Autodesk Fusion 360 part; units mm, degrees
note: some values were not read from the file. Set by a fixed rule: which sketch regions a step uses.
(part 3 of 5)
  spline S639 degree 3 poles (-6.513678, -34.419833) (-6.519277, -34.39743) (-6.526746, -34.375961) (-6.536703, -34.354802) knots 0 0 0 0 1 1 1 1
  spline S640 degree 3 poles (-6.536703, -34.354802) (-6.546349, -34.333955) (-6.557862, -34.314042) (-6.571552, -34.295373) knots 0 0 0 0 1 1 1 1
  spline S641 degree 3 poles (-6.571552, -34.295373) (-6.585243, -34.276704) (-6.600489, -34.25959) (-6.617603, -34.244033) knots 0 0 0 0 1 1 1 1
  spline S642 degree 3 poles (-6.617603, -34.244033) (-6.634404, -34.228475) (-6.652762, -34.214474) (-6.672365, -34.20265) knots 0 0 0 0 1 1 1 1
  spline S643 degree 3 poles (-6.672365, -34.20265) (-6.692279, -34.190515) (-6.712815, -34.180558) (-6.734595, -34.172779) knots 0 0 0 0 1 1 1 1
  spline S644 degree 3 poles (-6.734595, -34.172779) (-6.756065, -34.164689) (-6.778467, -34.159089) (-6.801181, -34.155355) knots 0 0 0 0 1 1 1 1
  spline S645 degree 3 poles (-6.801181, -34.155355) (-6.823895, -34.15193) (-6.84692, -34.150688) (-6.869946, -34.151619) knots 0 0 0 0 1 1 1 1
  spline S646 degree 3 poles (-6.869946, -34.151619) (-6.892971, -34.15255) (-6.915684, -34.155666) (-6.938087, -34.161264) knots 0 0 0 0 1 1 1 1
  spline S647 degree 3 poles (-6.938087, -34.161264) (-6.96049, -34.166554) (-6.98227, -34.174333) (-7.003117, -34.183978) knots 0 0 0 0 1 1 1 1
  spline S648 degree 3 poles (-7.003117, -34.183978) (-7.024276, -34.193624) (-7.043878, -34.205448) (-7.062547, -34.218827) knots 0 0 0 0 1 1 1 1
  spline S649 degree 3 poles (-7.062547, -34.218827) (-7.081217, -34.232518) (-7.098329, -34.247764) (-7.114198, -34.264877) knots 0 0 0 0 1 1 1 1
  spline S650 degree 3 poles (-7.114198, -34.264877) (-7.752679, -34.978656) (-8.346665, -35.728217) (-8.895845, -36.513561) knots 0 0 0 0 1 1 1 1
  spline S651 degree 3 poles (-8.895845, -36.513561) (-8.903935, -36.454753) (-8.912647, -36.395946) (-8.921671, -36.337761) knots 0 0 0 0 1 1 1 1
  line L13 (-8.921671, -36.337761) -> (-9.100893, -34.942252)
  spline S652 degree 3 poles (-9.100893, -34.942252) (-9.103697, -34.919227) (-9.108983, -34.896824) (-9.116451, -34.874732) knots 0 0 0 0 1 1 1 1
  spline S653 degree 3 poles (-9.116451, -34.874732) (-9.123604, -34.852951) (-9.132942, -34.831793) (-9.144454, -34.811569) knots 0 0 0 0 1 1 1 1
  spline S654 degree 3 poles (-9.144454, -34.811569) (-9.155967, -34.791655) (-9.169346, -34.772675) (-9.184593, -34.75525) knots 0 0 0 0 1 1 1 1
  spline S655 degree 3 poles (-9.184593, -34.75525) (-9.199528, -34.737826) (-9.21633, -34.721957) (-9.234688, -34.707955) knots 0 0 0 0 1 1 1 1
  spline S656 degree 3 poles (-9.234688, -34.707955) (-9.253046, -34.693643) (-9.272337, -34.681508) (-9.293184, -34.67124) knots 0 0 0 0 1 1 1 1
  spline S657 degree 3 poles (-9.293184, -34.67124) (-9.31372, -34.660972) (-9.335501, -34.652571) (-9.357592, -34.646659) knots 0 0 0 0 1 1 1 1
  spline S658 degree 3 poles (-9.357592, -34.646659) (-9.379995, -34.640438) (-9.402709, -34.636702) (-9.425734, -34.635146) knots 0 0 0 0 1 1 1 1
  spline S659 degree 3 poles (-9.425734, -34.635146) (-9.448759, -34.633593) (-9.471784, -34.634215) (-9.494809, -34.637322) knots 0 0 0 0 1 1 1 1
  spline S660 degree 3 poles (-9.494809, -34.637322) (-9.517835, -34.640125) (-9.540237, -34.645412) (-9.562018, -34.652568) knots 0 0 0 0 1 1 1 1
  spline S661 degree 3 poles (-9.562018, -34.652568) (-9.58411, -34.660031) (-9.604957, -34.669682) (-9.625181, -34.681194) knots 0 0 0 0 1 1 1 1
  spline S662 degree 3 poles (-9.625181, -34.681194) (-9.645095, -34.692707) (-9.663764, -34.706086) (-9.681189, -34.721332) knots 0 0 0 0 1 1 1 1
  spline S663 degree 3 poles (-9.681189, -34.721332) (-9.698613, -34.736268) (-9.714482, -34.75307) (-9.728483, -34.771428) knots 0 0 0 0 1 1 1 1
  spline S664 degree 3 poles (-9.728483, -34.771428) (-9.742796, -34.789786) (-9.754931, -34.809388) (-9.765199, -34.830235) knots 0 0 0 0 1 1 1 1
  spline S665 degree 3 poles (-9.765199, -34.830235) (-9.775467, -34.850771) (-9.783557, -34.872552) (-9.78978, -34.894954) knots 0 0 0 0 1 1 1 1
  spline S666 degree 3 poles (-9.78978, -34.894954) (-9.795691, -34.917046) (-9.799426, -34.93976) (-9.800981, -34.963096) knots 0 0 0 0 1 1 1 1
  spline S667 degree 3 poles (-9.800981, -34.963096) (-9.802535, -34.986121) (-9.801914, -35.009147) (-9.799117, -35.032172) knots 0 0 0 0 1 1 1 1
  line L14 (-9.799117, -35.032172) -> (-9.614915, -36.433597)
  spline S668 degree 3 poles (-12.713349, -48.832314) (-12.663254, -48.841337) (-12.617515, -48.860318) (-12.575511, -48.888943) knots 0 0 0 0 1 1 1 1
  spline S669 degree 3 poles (-12.575511, -48.888943) (-12.093538, -49.210362) (-11.58294, -49.476706) (-11.043407, -49.688288) knots 0 0 0 0 1 1 1 1
  spline S670 degree 3 poles (-11.043407, -49.688288) (-10.504181, -49.89956) (-9.948468, -50.05109) (-9.376574, -50.142879) knots 0 0 0 0 1 1 1 1
  spline S671 degree 3 poles (-9.376574, -50.142879) (-8.808723, -50.255515) (-8.234962, -50.305922) (-7.656535, -50.294098) knots 0 0 0 0 1 1 1 1
  spline S672 degree 3 poles (-7.656535, -50.294098) (-7.077172, -50.282586) (-6.5059, -50.209154) (-5.942718, -50.073493) knots 0 0 0 0 1 1 1 1
  spline S673 degree 3 poles (-5.943652, -50.073493) (-5.920315, -50.066961) (-5.89729, -50.062602) (-5.873954, -50.060735) knots 0 0 0 0 1 1 1 1
  spline S674 degree 3 poles (-5.874575, -50.060738) (-5.850306, -50.058871) (-5.82697, -50.059182) (-5.803634, -50.061978) knots 0 0 0 0 1 1 1 1
  spline S675 degree 3 poles (-5.804566, -50.061669) (-5.780297, -50.06478) (-5.757583, -50.069759) (-5.73518, -50.076913) knots 0 0 0 0 1 1 1 1
  spline S676 degree 3 poles (-5.735802, -50.076915) (-5.712777, -50.084376) (-5.69162, -50.093715) (-5.671083, -50.105227) knots 0 0 0 0 1 1 1 1
  spline S677 degree 3 poles (-5.671705, -50.10523) (-5.650547, -50.117051) (-5.631567, -50.130431) (-5.613831, -50.145988) knots 0 0 0 0 1 1 1 1
  spline S678 degree 3 poles (-5.614454, -50.145991) (-5.596096, -50.161546) (-5.580228, -50.178348) (-5.565914, -50.197017) knots 0 0 0 0 1 1 1 1
  spline S679 degree 3 poles (-5.566536, -50.197019) (-5.551601, -50.215686) (-5.539155, -50.235599) (-5.528887, -50.256758) knots 0 0 0 0 1 1 1 1
  spline S680 degree 3 poles (-5.529509, -50.25676) (-5.518619, -50.277916) (-5.510529, -50.300008) (-5.504618, -50.322721) knots 0 0 0 0 1 1 1 1
  spline S681 degree 3 poles (-5.505239, -50.322724) (-5.498707, -50.345435) (-5.494972, -50.368461) (-5.493727, -50.392108) knots 0 0 0 0 1 1 1 1
  spline S682 degree 3 poles (-5.494349, -50.39211) (-5.492485, -50.415755) (-5.493409, -50.439092) (-5.496842, -50.462428) knots 0 0 0 0 1 1 1 1
  spline S683 degree 3 poles (-5.497464, -50.462119) (-5.500267, -50.485453) (-5.505866, -50.508167) (-5.513956, -50.53057) knots 0 0 0 0 1 1 1 1
  spline S684 degree 3 poles (-5.514577, -50.530261) (-5.521738, -50.552662) (-5.532002, -50.57382) (-5.544137, -50.593733) knots 0 0 0 0 1 1 1 1
  spline S685 degree 3 poles (-5.544758, -50.593736) (-5.556272, -50.613958) (-5.570274, -50.632627) (-5.586143, -50.650052) knots 0 0 0 0 1 1 1 1
  spline S686 degree 3 poles (-5.587075, -50.650054) (-5.602322, -50.667476) (-5.619746, -50.683034) (-5.638726, -50.696724) knots 0 0 0 0 1 1 1 1
  spline S687 degree 3 poles (-5.639348, -50.696415) (-5.657707, -50.710415) (-5.677931, -50.722238) (-5.699401, -50.731884) knots 0 0 0 0 1 1 1 1
  spline S688 degree 3 poles (-5.700022, -50.731887) (-5.72087, -50.741841) (-5.742962, -50.749309) (-5.765987, -50.754598) knots 0 0 0 0 1 1 1 1
  spline S689 degree 3 poles (-5.766608, -50.754289) (-6.378019, -50.903017) (-6.999075, -50.984227) (-7.628844, -50.997918) knots 0 0 0 0 1 1 1 1
  spline S690 degree 3 poles (-7.629154, -50.997609) (-8.258612, -51.011608) (-8.882468, -50.957779) (-9.500411, -50.836122) knots 0 0 0 0 1 1 1 1
  spline S691 degree 3 poles (-9.500411, -50.836122) (-10.12178, -50.735618) (-10.7251, -50.570086) (-11.310995, -50.339526) knots 0 0 0 0 1 1 1 1
  spline S692 degree 3 poles (-11.310995, -50.339526) (-11.896892, -50.108961) (-12.451362, -49.818658) (-12.974716, -49.468616) knots 0 0 0 0 1 1 1 1
  spline S693 degree 3 poles (-12.974716, -49.468616) (-13.007699, -49.4459) (-13.036013, -49.418208) (-13.059661, -49.385537) knots 0 0 0 0 1 1 1 1
  spline S694 degree 3 poles (-13.059661, -49.385537) (-13.082996, -49.353177) (-13.10042, -49.317706) (-13.111934, -49.279123) knots 0 0 0 0 1 1 1 1
  spline S695 degree 3 poles (-13.111934, -49.279123) (-13.123447, -49.240541) (-13.128114, -49.201336) (-13.125936, -49.161197) knots 0 0 0 0 1 1 1 1
  spline S696 degree 3 poles (-13.125936, -49.161197) (-13.124071, -49.121059) (-13.115357, -49.082165) (-13.10011, -49.045138) knots 0 0 0 0 1 1 1 1
  spline S697 degree 3 poles (-13.10011, -49.045138) (-13.084864, -49.008112) (-13.063706, -48.974507) (-13.036947, -48.944326) knots 0 0 0 0 1 1 1 1
  spline S698 degree 3 poles (-13.036947, -48.944326) (-13.010188, -48.914455) (-12.979384, -48.889874) (-12.944224, -48.870583) knots 0 0 0 0 1 1 1 1
  spline S699 degree 3 poles (-12.944224, -48.870583) (-12.909064, -48.850981) (-12.871415, -48.838223) (-12.831899, -48.831689) knots 0 0 0 0 1 1 1 1
  spline S700 degree 3 poles (-12.831899, -48.831689) (-12.792383, -48.825158) (-12.752867, -48.825158) (-12.713349, -48.832314) knots 0 0 0 0 1 1 1 1
  spline S701 degree 3 poles (-13.602617, -45.813223) (-13.50616, -45.830336) (-13.43024, -45.879498) (-13.374544, -45.959782) knots 0 0 0 0 1 1 1 1
  spline S702 degree 3 poles (-13.374544, -45.959782) (-13.314803, -46.051253) (-13.252573, -46.140553) (-13.188165, -46.228608) knots 0 0 0 0 1 1 1 1
  spline S703 degree 3 poles (-13.187853, -46.227682) (-13.123445, -46.316353) (-13.056859, -46.402541) (-12.988095, -46.486863) knots 0 0 0 0 1 1 1 1
  spline S704 degree 3 poles (-12.988095, -46.486248) (-12.919331, -46.571185) (-12.848388, -46.653951) (-12.775268, -46.73485) knots 0 0 0 0 1 1 1 1
  spline S705 degree 3 poles (-12.775268, -46.733924) (-12.702148, -46.815438) (-12.627161, -46.89447) (-12.550307, -46.971324) knots 0 0 0 0 1 1 1 1
  spline S706 degree 3 poles (-12.549995, -46.970709) (-12.473141, -47.048489) (-12.394109, -47.123477) (-12.313521, -47.196597) knots 0 0 0 0 1 1 1 1
  spline S707 degree 3 poles (-12.31321, -47.195671) (-12.232622, -47.269406) (-12.149856, -47.340348) (-12.065534, -47.409113) knots 0 0 0 0 1 1 1 1
  spline S708 degree 3 poles (-12.065534, -47.408498) (-11.981213, -47.477877) (-11.895024, -47.544774) (-11.80728, -47.609182) knots 0 0 0 0 1 1 1 1
  spline S709 degree 3 poles (-11.80728, -47.608256) (-11.719535, -47.67359) (-11.630235, -47.73582) (-11.539068, -47.795561) knots 0 0 0 0 1 1 1 1
  spline S710 degree 3 poles (-11.539068, -47.794946) (-11.448212, -47.855613) (-11.355801, -47.913176) (-11.261833, -47.96825) knots 0 0 0 0 1 1 1 1
  spline S711 degree 3 poles (-11.261833, -47.967635) (-11.168177, -48.023323) (-11.072965, -48.076219) (-10.976508, -48.126625) knots 0 0 0 0 1 1 1 1
  spline S712 degree 3 poles (-10.976197, -48.12601) (-10.879741, -48.177032) (-10.782039, -48.224949) (-10.683094, -48.270377) knots 0 0 0 0 1 1 1 1
  spline S713 degree 3 poles (-10.683094, -48.269762) (-10.584148, -48.315805) (-10.484269, -48.358743) (-10.383145, -48.398882) knots 0 0 0 0 1 1 1 1
  spline S714 degree 3 poles (-10.382834, -48.398267) (-10.282021, -48.439331) (-10.179964, -48.47698) (-10.076973, -48.51214) knots 0 0 0 0 1 1 1 1
  spline S715 degree 3 poles (-10.076662, -48.511525) (-9.973671, -48.5473) (-9.870058, -48.579971) (-9.7652, -48.609842) knots 0 0 0 0 1 1 1 1
  spline S716 degree 3 poles (-9.7652, -48.609227) (-9.660654, -48.639712) (-9.555174, -48.666782) (-9.449072, -48.691363) knots 0 0 0 0 1 1 1 1
  spline S717 degree 3 poles (-9.449072, -48.690748) (-9.342969, -48.715944) (-9.236556, -48.737724) (-9.129209, -48.757016) knots 0 0 0 0 1 1 1 1
  spline S718 degree 3 poles (-9.129209, -48.75609) (-9.022173, -48.775996) (-8.914515, -48.792487) (-8.806545, -48.806177) knots 0 0 0 0 1 1 1 1
  spline S719 degree 3 poles (-8.806235, -48.805562) (-8.698577, -48.819868) (-8.590296, -48.830758) (-8.481704, -48.838848) knots 0 0 0 0 1 1 1 1
  spline S720 degree 3 poles (-8.481394, -48.838233) (-8.373113, -48.846938) (-8.26421, -48.852539) (-8.155619, -48.855028) knots 0 0 0 0 1 1 1 1
  spline S721 degree 3 poles (-8.155309, -48.854413) (-8.046716, -48.857831) (-7.937813, -48.857512) (-7.828911, -48.85471) knots 0 0 0 0 1 1 1 1
  spline S722 degree 3 poles (-7.828912, -48.854095) (-7.720008, -48.851914) (-7.611417, -48.846309) (-7.502825, -48.837907) knots 0 0 0 0 1 1 1 1
  spline S723 degree 3 poles (-7.502827, -48.837292) (-7.394234, -48.829506) (-7.285954, -48.818305) (-7.177984, -48.804614) knots 0 0 0 0 1 1 1 1
  spline S724 degree 3 poles (-7.177985, -48.803688) (-7.070015, -48.790613) (-6.962357, -48.774122) (-6.855321, -48.75483) knots 0 0 0 0 1 1 1 1
  spline S725 degree 3 poles (-6.855322, -48.753904) (-6.748285, -48.735228) (-6.641561, -48.713447) (-6.535459, -48.688555) knots 0 0 0 0 1 1 1 1
  spline S726 degree 3 poles (-6.53546, -48.68794) (-6.429357, -48.663974) (-6.324187, -48.636282) (-6.21933, -48.606412) knots 0 0 0 0 1 1 1 1
  spline S727 degree 3 poles (-6.219332, -48.605797) (-6.114784, -48.57623) (-6.01086, -48.543559) (-5.907869, -48.508088) knots 0 0 0 0 1 1 1 1
  spline S728 degree 3 poles (-5.90787, -48.507473) (-5.804878, -48.472928) (-5.702821, -48.434968) (-5.601697, -48.394207) knots 0 0 0 0 1 1 1 1
  spline S729 degree 3 poles (-5.601698, -48.393592) (-5.500885, -48.353758) (-5.400694, -48.310819) (-5.301749, -48.26508) knots 0 0 0 0 1 1 1 1
  spline S730 degree 3 poles (-5.30175, -48.264465) (-5.202803, -48.219341) (-5.105101, -48.171424) (-5.008645, -48.120706) knots 0 0 0 0 1 1 1 1
  spline S731 degree 3 poles (-5.008646, -48.120091) (-4.912188, -48.0703) (-4.817287, -48.017404) (-4.72332, -47.962019) knots 0 0 0 0 1 1 1 1
  spline S732 degree 3 poles (-4.723321, -47.961093) (-4.629664, -47.906635) (-4.537252, -47.848761) (-4.446396, -47.788709) knots 0 0 0 0 1 1 1 1
  spline S733 degree 3 poles (-4.446086, -47.788094) (-4.35554, -47.728657) (-4.26624, -47.666115) (-4.178496, -47.601707) knots 0 0 0 0 1 1 1 1
  spline S734 degree 3 poles (-4.178186, -47.601092) (-4.140535, -47.578371) (-4.099463, -47.562814) (-4.055591, -47.555035) knots 0 0 0 0 1 1 1 1
  spline S735 degree 3 poles (-4.055278, -47.554425) (-4.011719, -47.547254) (-3.967847, -47.547874) (-3.924286, -47.556899) knots 0 0 0 0 1 1 1 1
  spline S736 degree 3 poles (-3.923972, -47.556289) (-3.880414, -47.565923) (-3.839964, -47.582414) (-3.802626, -47.606994) knots 0 0 0 0 1 1 1 1
  spline S737 degree 3 poles (-3.802624, -47.606384) (-3.765288, -47.631264) (-3.733862, -47.661757) (-3.708036, -47.698162) knots 0 0 0 0 1 1 1 1
  spline S738 degree 3 poles (-3.708034, -47.697551) (-3.682211, -47.734566) (-3.664164, -47.774393) (-3.653585, -47.817643) knots 0 0 0 0 1 1 1 1
  spline S739 degree 3 poles (-3.653272, -47.817033) (-3.642695, -47.861204) (-3.640517, -47.905076) (-3.646429, -47.94926) knots 0 0 0 0 1 1 1 1
  spline S740 degree 3 poles (-3.646426, -47.948339) (-3.652652, -47.993443) (-3.666653, -48.034826) (-3.688434, -48.074031) knots 0 0 0 0 1 1 1 1
  spline S741 degree 3 poles (-3.68812, -48.07311) (-3.710214, -48.112925) (-3.738218, -48.146529) (-3.773067, -48.174533) knots 0 0 0 0 1 1 1 1
  spline S742 degree 3 poles (-3.772753, -48.173922) (-3.870146, -48.245786) (-3.969092, -48.314861) (-4.069593, -48.381136) knots 0 0 0 0 1 1 1 1
  spline S743 degree 3 poles (-4.069591, -48.380526) (-4.170406, -48.447411) (-4.272774, -48.511197) (-4.376698, -48.572183) knots 0 0 0 0 1 1 1 1
  spline S744 degree 3 poles (-4.376385, -48.571573) (-4.480623, -48.633479) (-4.585791, -48.691976) (-4.692827, -48.747671) knots 0 0 0 0 1 1 1 1
  spline S745 degree 3 poles (-4.692514, -48.747061) (-4.799552, -48.803367) (-4.907832, -48.856574) (-5.017357, -48.90698) knots 0 0 0 0 1 1 1 1
  spline S746 degree 3 poles (-5.017043, -48.90637) (-5.126882, -48.957387) (-5.237339, -49.004682) (-5.349354, -49.049487) knots 0 0 0 0 1 1 1 1
  spline S747 degree 3 poles (-5.349352, -49.048877) (-5.461368, -49.094293) (-5.574315, -49.135987) (-5.688197, -49.175192) knots 0 0 0 0 1 1 1 1
  spline S748 degree 3 poles (-5.688195, -49.174271) (-5.802389, -49.214086) (-5.917203, -49.250179) (-6.033263, -49.283472) knots 0 0 0 0 1 1 1 1
  spline S749 degree 3 poles (-6.032949, -49.282862) (-6.14901, -49.316454) (-6.265692, -49.346947) (-6.382995, -49.374017) knots 0 0 0 0 1 1 1 1
  spline S750 degree 3 poles (-6.382993, -49.373407) (-6.500299, -49.401398) (-6.618225, -49.425668) (-6.737084, -49.447137) knots 0 0 0 0 1 1 1 1
  spline S751 degree 3 poles (-6.736771, -49.446216) (-6.855633, -49.468296) (-6.974492, -49.486653) (-7.093974, -49.5019) knots 0 0 0 0 1 1 1 1
  spline S752 degree 3 poles (-7.093972, -49.50129) (-7.213766, -49.517146) (-7.33356, -49.529281) (-7.453664, -49.538615) knots 0 0 0 0 1 1 1 1
  spline S753 degree 3 poles (-7.45335, -49.538005) (-7.573768, -49.54795) (-7.694183, -49.553862) (-7.814598, -49.556973) knots 0 0 0 0 1 1 1 1
  spline S754 degree 3 poles (-7.814284, -49.556363) (-7.935013, -49.560087) (-8.055428, -49.560398) (-8.175843, -49.557292) knots 0 0 0 0 1 1 1 1
  spline S755 degree 3 poles (-8.17553, -49.556682) (-8.296257, -49.554489) (-8.416674, -49.548268) (-8.536778, -49.539245) knots 0 0 0 0 1 1 1 1
  spline S756 degree 3 poles (-8.536464, -49.538635) (-8.656882, -49.530222) (-8.776673, -49.518087) (-8.896155, -49.50284) knots 0 0 0 0 1 1 1 1
  spline S757 degree 3 poles (-8.896154, -49.50223) (-9.015637, -49.487905) (-9.134807, -49.469547) (-9.253356, -49.448389) knots 0 0 0 0 1 1 1 1
  spline S758 degree 3 poles (-9.253354, -49.447779) (-9.371904, -49.427231) (-9.48983, -49.403272) (-9.607445, -49.375891) knots 0 0 0 0 1 1 1 1
  spline S759 degree 3 poles (-9.607132, -49.375281) (-9.724748, -49.348821) (-9.84143, -49.31864) (-9.957178, -49.285658) knots 0 0 0 0 1 1 1 1
  spline S760 degree 3 poles (-9.957176, -49.285047) (-10.072925, -49.252676) (-10.188051, -49.216582) (-10.301932, -49.178) knots 0 0 0 0 1 1 1 1
  spline S761 degree 3 poles (-10.301931, -49.177078) (-10.416124, -49.139106) (-10.529072, -49.097101) (-10.641086, -49.052606) knots 0 0 0 0 1 1 1 1
  spline S762 degree 3 poles (-10.640774, -49.051996) (-10.752789, -49.008112) (-10.863558, -48.960817) (-10.973083, -48.91041) knots 0 0 0 0 1 1 1 1
  spline S763 degree 3 poles (-10.973082, -48.9098) (-11.082608, -48.860315) (-11.190888, -48.80742) (-11.297613, -48.751724) knots 0 0 0 0 1 1 1 1
  spline S764 degree 3 poles (-11.297612, -48.750802) (-11.404649, -48.696028) (-11.510129, -48.637532) (-11.614053, -48.576546) knots 0 0 0 0 1 1 1 1
  spline S765 degree 3 poles (-11.613741, -48.575936) (-11.717666, -48.515561) (-11.820034, -48.452086) (-11.920847, -48.385811) knots 0 0 0 0 1 1 1 1
  spline S766 degree 3 poles (-11.920535, -48.385201) (-12.021349, -48.319536) (-12.120294, -48.250772) (-12.217684, -48.179518) knots 0 0 0 0 1 1 1 1
  spline S767 degree 3 poles (-12.217683, -48.178908) (-12.314763, -48.108265) (-12.410286, -48.034833) (-12.503632, -47.958602) knots 0 0 0 0 1 1 1 1
  spline S768 degree 3 poles (-12.50363, -47.957991) (-12.597288, -47.882681) (-12.688766, -47.804271) (-12.778377, -47.723683) knots 0 0 0 0 1 1 1 1
  spline S769 degree 3 poles (-12.778065, -47.723073) (-12.867677, -47.643095) (-12.955111, -47.560018) (-13.040676, -47.475074) knots 0 0 0 0 1 1 1 1
  spline S770 degree 3 poles (-13.040365, -47.474153) (-13.125931, -47.389819) (-13.209009, -47.302697) (-13.289907, -47.213397) knots 0 0 0 0 1 1 1 1
  spline S771 degree 3 poles (-13.289907, -47.212475) (-13.371117, -47.124097) (-13.449527, -47.032618) (-13.52607, -46.939273) knots 0 0 0 0 1 1 1 1
  spline S772 degree 3 poles (-13.525759, -46.938663) (-13.602303, -46.845928) (-13.676045, -46.750716) (-13.747609, -46.653948) knots 0 0 0 0 1 1 1 1
  spline S773 degree 3 poles (-13.747609, -46.653027) (-13.819174, -46.55687) (-13.888249, -46.457924) (-13.954835, -46.357422) knots 0 0 0 0 1 1 1 1
  spline S774 degree 3 poles (-13.954524, -46.356812) (-13.974127, -46.328796) (-13.989062, -46.297993) (-13.99933, -46.265011) knots 0 0 0 0 1 1 1 1
  spline S775 degree 3 poles (-13.99933, -46.265011) (-14.009598, -46.232029) (-14.014887, -46.198113) (-14.015198, -46.163576) knots 0 0 0 0 1 1 1 1
  spline S776 degree 3 poles (-14.015198, -46.163576) (-14.015835, -46.129038) (-14.011152, -46.095123) (-14.001508, -46.061829) knots 0 0 0 0 1 1 1 1
  spline S777 degree 3 poles (-14.001508, -46.061829) (-13.991862, -46.028536) (-13.977549, -45.997421) (-13.95888, -45.968484) knots 0 0 0 0 1 1 1 1
  spline S778 degree 3 poles (-13.95888, -45.968484) (-13.9399, -45.939547) (-13.917497, -45.913722) (-13.891049, -45.891319) knots 0 0 0 0 1 1 1 1
  spline S779 degree 3 poles (-13.891049, -45.891319) (-13.864913, -45.868916) (-13.835665, -45.85087) (-13.804239, -45.837179) knots 0 0 0 0 1 1 1 1
  spline S780 degree 3 poles (-13.804239, -45.837179) (-13.772501, -45.823177) (-13.739519, -45.814465) (-13.705293, -45.810109) knots 0 0 0 0 1 1 1 1
  spline S781 degree 3 poles (-13.705293, -45.810109) (-13.670755, -45.806061) (-13.63684, -45.806995) (-13.602617, -45.813223) knots 0 0 0 0 1 1 1 1
  spline S782 degree 3 poles (-13.428991, -40.838231) (-13.406281, -40.842288) (-13.384189, -40.848509) (-13.362716, -40.8569) knots 0 0 0 0 1 1 1 1
  spline S783 degree 3 poles (-13.362716, -40.8569) (-13.341251, -40.865311) (-13.320715, -40.87589) (-13.301109, -40.888326) knots 0 0 0 0 1 1 1 1
  spline S784 degree 3 poles (-13.301109, -40.888326) (-13.281821, -40.900782) (-13.263774, -40.915095) (-13.246968, -40.930954) knots 0 0 0 0 1 1 1 1
  spline S785 degree 3 poles (-13.246968, -40.930954) (-13.230481, -40.946832) (-13.215546, -40.964568) (-13.202474, -40.983538) knots 0 0 0 0 1 1 1 1
  spline S786 degree 3 poles (-13.202474, -40.983538) (-13.189099, -41.002217) (-13.177897, -41.022442) (-13.168558, -41.04359) knots 0 0 0 0 1 1 1 1
  spline S787 degree 3 poles (-13.168558, -41.04359) (-13.159539, -41.064758) (-13.152382, -41.086539) (-13.1474, -41.109243) knots 0 0 0 0 1 1 1 1
  spline S788 degree 3 poles (-13.1474, -41.109243) (-13.142426, -41.131656) (-13.139622, -41.154681) (-13.13931, -41.177696) knots 0 0 0 0 1 1 1 1
  spline S789 degree 3 poles (-13.13931, -41.177696) (-13.138996, -41.200731) (-13.140556, -41.223756) (-13.1446, -41.24646) knots 0 0 0 0 1 1 1 1
  spline S790 degree 3 poles (-13.1446, -41.24646) (-13.162339, -41.345105) (-13.176963, -41.444362) (-13.188783, -41.543609) knots 0 0 0 0 1 1 1 1
  spline S791 degree 3 poles (-13.188783, -41.543609) (-13.200611, -41.643187) (-13.209634, -41.742755) (-13.215542, -41.842624) knots 0 0 0 0 1 1 1 1
  spline S792 degree 3 poles (-13.215542, -41.842624) (-13.222078, -41.942824) (-13.225503, -42.043015) (-13.226125, -42.143205) knots 0 0 0 0 1 1 1 1
  spline S793 degree 3 poles (-13.22581, -42.142573) (-13.226443, -42.243396) (-13.22426, -42.343275) (-13.218972, -42.443465) knots 0 0 0 0 1 1 1 1
  spline S794 degree 3 poles (-13.218657, -42.442833) (-13.213994, -42.543344) (-13.205904, -42.643224) (-13.195012, -42.742792) knots 0 0 0 0 1 1 1 1
  spline S795 degree 3 poles (-13.194699, -42.741849) (-13.184123, -42.84236) (-13.170743, -42.941617) (-13.154253, -43.040563) knots 0 0 0 0 1 1 1 1
  spline S796 degree 3 poles (-13.154253, -43.040563) (-13.137761, -43.139197) (-13.118471, -43.237521) (-13.096379, -43.335222) knots 0 0 0 0 1 1 1 1
  spline S797 degree 3 poles (-13.096379, -43.335222) (-13.074287, -43.432923) (-13.049706, -43.530002) (-13.022014, -43.626147) knots 0 0 0 0 1 1 1 1
  spline S798 degree 3 poles (-13.022014, -43.626147) (-12.994322, -43.722604) (-12.96414, -43.817816) (-12.931158, -43.912406) knots 0 0 0 0 1 1 1 1
  spline S799 degree 3 poles (-12.931158, -43.912406) (-12.898176, -44.006995) (-12.862705, -44.100652) (-12.824434, -44.193063) knots 0 0 0 0 1 1 1 1
  spline S800 degree 3 poles (-12.824434, -44.193063) (-12.786162, -44.285786) (-12.74509, -44.376953) (-12.70184, -44.467187) knots 0 0 0 0 1 1 1 1
  spline S801 degree 3 poles (-12.70184, -44.467187) (-12.658279, -44.55742) (-12.612229, -44.646409) (-12.56369, -44.733842) knots 0 0 0 0 1 1 1 1
  spline S802 degree 3 poles (-12.56369, -44.733842) (-12.51515, -44.821587) (-12.464433, -44.907775) (-12.410915, -44.992408) knots 0 0 0 0 1 1 1 1
  spline S803 degree 3 poles (-12.410915, -44.992408) (-12.357397, -45.077041) (-12.301701, -45.160118) (-12.243516, -45.24164) knots 0 0 0 0 1 1 1 1
  spline S804 degree 3 poles (-12.243516, -45.24164) (-12.185642, -45.323161) (-12.124968, -45.402816) (-12.062427, -45.480914) knots 0 0 0 0 1 1 1 1
  spline S805 degree 3 poles (-12.062427, -45.480914) (-11.999885, -45.559013) (-11.934855, -45.635245) (-11.867958, -45.70961) knots 0 0 0 0 1 1 1 1
  spline S806 degree 3 poles (-11.867958, -45.70961) (-11.80106, -45.783975) (-11.731985, -45.856473) (-11.660731, -45.926793) knots 0 0 0 0 1 1 1 1
  spline S807 degree 3 poles (-11.660731, -45.926793) (-11.589789, -45.997113) (-11.516669, -46.065566) (-11.441682, -46.131841) knots 0 0 0 0 1 1 1 1
  spline S808 degree 3 poles (-11.441682, -46.131841) (-11.366694, -46.198116) (-11.28984, -46.262213) (-11.21143, -46.324132) knots 0 0 0 0 1 1 1 1
  spline S809 degree 3 poles (-11.21143, -46.324132) (-11.132709, -46.38605) (-11.052433, -46.445791) (-10.970289, -46.503043) knots 0 0 0 0 1 1 1 1
  spline S810 degree 3 poles (-10.970289, -46.503043) (-10.888456, -46.560295) (-10.804757, -46.615368) (-10.719813, -46.667953) knots 0 0 0 0 1 1 1 1
  spline S811 degree 3 poles (-10.719813, -46.667953) (-10.634558, -46.720537) (-10.548058, -46.770632) (-10.460003, -46.818238) knots 0 0 0 0 1 1 1 1
  spline S812 degree 3 poles (-10.460003, -46.818238) (-10.371947, -46.865844) (-10.282647, -46.910961) (-10.192102, -46.953589) knots 0 0 0 0 1 1 1 1
  spline S813 degree 3 poles (-10.192102, -46.953589) (-10.101557, -46.996216) (-10.010079, -47.036043) (-9.917045, -47.073381) knots 0 0 0 0 1 1 1 1
  spline S814 degree 3 poles (-9.917045, -47.073381) (-9.824322, -47.11072) (-9.730666, -47.145257) (-9.635765, -47.177306) knots 0 0 0 0 1 1 1 1
  spline S815 degree 3 poles (-9.635765, -47.177306) (-9.540865, -47.209354) (-9.445341, -47.238602) (-9.348885, -47.265361) knots 0 0 0 0 1 1 1 1
  spline S816 degree 3 poles (-9.348885, -47.265361) (-9.252428, -47.291809) (-9.155349, -47.315456) (-9.057648, -47.336615) knots 0 0 0 0 1 1 1 1
  spline S817 degree 3 poles (-9.057648, -47.336615) (-8.959636, -47.357773) (-8.861312, -47.37582) (-8.762678, -47.391377) knots 0 0 0 0 1 1 1 1
  spline S818 degree 3 poles (-8.762678, -47.391377) (-8.663732, -47.406623) (-8.564475, -47.419381) (-8.464907, -47.429026) knots 0 0 0 0 1 1 1 1
  spline S819 degree 3 poles (-8.464907, -47.429026) (-8.365339, -47.438983) (-8.265771, -47.445828) (-8.16558, -47.449873) knots 0 0 0 0 1 1 1 1
  spline S820 degree 3 poles (-8.16558, -47.449873) (-8.065701, -47.453921) (-7.965822, -47.455474) (-7.865631, -47.45361) knots 0 0 0 0 1 1 1 1
  spline S821 degree 3 poles (-7.865631, -47.45361) (-7.765752, -47.452056) (-7.665873, -47.4477) (-7.565995, -47.440541) knots 0 0 0 0 1 1 1 1
  spline S822 degree 3 poles (-7.565995, -47.440541) (-7.542659, -47.438358) (-7.519322, -47.438358) (-7.495986, -47.44086) knots 0 0 0 0 1 1 1 1
  spline S823 degree 3 poles (-7.495986, -47.44086) (-7.47265, -47.443344) (-7.449936, -47.448021) (-7.427533, -47.454861) knots 0 0 0 0 1 1 1 1
  spline S824 degree 3 poles (-7.427533, -47.454861) (-7.405441, -47.462023) (-7.383973, -47.471041) (-7.363437, -47.482243) knots 0 0 0 0 1 1 1 1
  spline S825 degree 3 poles (-7.363437, -47.482243) (-7.342901, -47.493755) (-7.323609, -47.506824) (-7.305874, -47.52207) knots 0 0 0 0 1 1 1 1
  spline S826 degree 3 poles (-7.305874, -47.52207) (-7.287827, -47.537005) (-7.271647, -47.553807) (-7.257023, -47.572165) knots 0 0 0 0 1 1 1 1
  spline S827 degree 3 poles (-7.257023, -47.572165) (-7.24271, -47.590834) (-7.229953, -47.610437) (-7.219374, -47.631284) knots 0 0 0 0 1 1 1 1
  spline S828 degree 3 poles (-7.219374, -47.631284) (-7.208795, -47.652131) (-7.200394, -47.673911) (-7.194172, -47.696314) knots 0 0 0 0 1 1 1 1
  spline S829 degree 3 poles (-7.194172, -47.696314) (-7.18795, -47.719028) (-7.183904, -47.742053) (-7.182036, -47.765389) knots 0 0 0 0 1 1 1 1
  spline S830 degree 3 poles (-7.182036, -47.765389) (-7.180483, -47.788726) (-7.181104, -47.812062) (-7.18421, -47.835398) knots 0 0 0 0 1 1 1 1
  spline S831 degree 3 poles (-7.18421, -47.835398) (-7.187014, -47.858735) (-7.1923, -47.881448) (-7.199768, -47.90354) knots 0 0 0 0 1 1 1 1
  spline S832 degree 3 poles (-7.199768, -47.90354) (-7.207231, -47.925943) (-7.216881, -47.947101) (-7.228705, -47.967326) knots 0 0 0 0 1 1 1 1
  spline S833 degree 3 poles (-7.228705, -47.967326) (-7.240529, -47.987551) (-7.254219, -48.006531) (-7.269777, -48.024266) knots 0 0 0 0 1 1 1 1
  spline S834 degree 3 poles (-7.269777, -48.024266) (-7.285335, -48.041691) (-7.302448, -48.05756) (-7.321117, -48.071561) knots 0 0 0 0 1 1 1 1
  spline S835 degree 3 poles (-7.321117, -48.071561) (-7.339786, -48.085874) (-7.359699, -48.098009) (-7.380858, -48.107966) knots 0 0 0 0 1 1 1 1
  spline S836 degree 3 poles (-7.380858, -48.107966) (-7.401705, -48.118234) (-7.423797, -48.126324) (-7.446511, -48.131924) knots 0 0 0 0 1 1 1 1
  spline S837 degree 3 poles (-7.446511, -48.131924) (-7.469225, -48.137834) (-7.492249, -48.141259) (-7.515586, -48.142504) knots 0 0 0 0 1 1 1 1
  spline S838 degree 3 poles (-7.515586, -48.142504) (-7.628845, -48.150593) (-7.741792, -48.155572) (-7.855362, -48.157439) knots 0 0 0 0 1 1 1 1
  spline S839 degree 3 poles (-7.855362, -48.157439) (-7.968621, -48.159303) (-8.08188, -48.158076) (-8.195138, -48.153391) knots 0 0 0 0 1 1 1 1
  spline S840 degree 3 poles (-8.195138, -48.153391) (-8.308397, -48.148724) (-8.421656, -48.140945) (-8.534292, -48.129744) knots 0 0 0 0 1 1 1 1
  spline S841 degree 3 poles (-8.534292, -48.129744) (-8.647239, -48.118854) (-8.759565, -48.104541) (-8.871579, -48.087116) knots 0 0 0 0 1 1 1 1
  spline S842 degree 3 poles (-8.871579, -48.087116) (-8.983593, -48.069381) (-9.095296, -48.048845) (-9.206066, -48.025197) knots 0 0 0 0 1 1 1 1
  spline S843 degree 3 poles (-9.206066, -48.025197) (-9.316835, -48.001239) (-9.426982, -47.974169) (-9.536196, -47.944298) knots 0 0 0 0 1 1 1 1
  spline S844 degree 3 poles (-9.536196, -47.944298) (-9.64541, -47.914117) (-9.754001, -47.880824) (-9.861348, -47.84473) knots 0 0 0 0 1 1 1 1
  spline S845 degree 3 poles (-9.861348, -47.84473) (-9.968695, -47.808326) (-10.075108, -47.769121) (-10.180277, -47.726804) knots 0 0 0 0 1 1 1 1
  spline S846 degree 3 poles (-10.180277, -47.726804) (-10.285446, -47.684488) (-10.38937, -47.639371) (-10.49205, -47.591143) knots 0 0 0 0 1 1 1 1
  spline S847 degree 3 poles (-10.49205, -47.591143) (-10.594729, -47.542915) (-10.695853, -47.491575) (-10.795421, -47.437746) knots 0 0 0 0 1 1 1 1
  spline S848 degree 3 poles (-10.795421, -47.437746) (-10.895301, -47.383606) (-10.993313, -47.326976) (-11.08977, -47.267235) knots 0 0 0 0 1 1 1 1
  spline S849 degree 3 poles (-11.08977, -47.267235) (-11.186226, -47.207806) (-11.280816, -47.145576) (-11.37385, -47.080545) knots 0 0 0 0 1 1 1 1
  spline S850 degree 3 poles (-11.37385, -47.080545) (-11.466884, -47.015515) (-11.55774, -46.947995) (-11.64704, -46.877675) knots 0 0 0 0 1 1 1 1
  spline S851 degree 3 poles (-11.64704, -46.877675) (-11.736029, -46.807666) (-11.823151, -46.735168) (-11.908095, -46.65987) knots 0 0 0 0 1 1 1 1
  spline S852 degree 3 poles (-11.908095, -46.65987) (-11.993039, -46.584883) (-12.075805, -46.507406) (-12.156393, -46.427441) knots 0 0 0 0 1 1 1 1
  spline S853 degree 3 poles (-12.156393, -46.427441) (-12.236981, -46.347475) (-12.315079, -46.265643) (-12.391, -46.181321) knots 0 0 0 0 1 1 1 1
  spline S854 degree 3 poles (-12.391, -46.181321) (-12.466921, -46.096999) (-12.540352, -46.010499) (-12.611607, -45.922133) knots 0 0 0 0 1 1 1 1
  spline S855 degree 3 poles (-12.611607, -45.922133) (-12.682549, -45.833766) (-12.751002, -45.743221) (-12.816654, -45.65081) knots 0 0 0 0 1 1 1 1
  spline S856 degree 3 poles (-12.816654, -45.65081) (-12.882617, -45.558398) (-12.945781, -45.464431) (-13.006455, -45.368285) knots 0 0 0 0 1 1 1 1
  spline S857 degree 3 poles (-13.006455, -45.368285) (-13.066818, -45.272451) (-13.124692, -45.17475) (-13.179455, -45.075493) knots 0 0 0 0 1 1 1 1
  spline S858 degree 3 poles (-13.179455, -45.075493) (-13.234528, -44.976236) (-13.286491, -44.875423) (-13.335963, -44.773055) knots 0 0 0 0 1 1 1 1
  spline S859 degree 3 poles (-13.335963, -44.773055) (-13.385125, -44.670997) (-13.431485, -44.567384) (-13.474736, -44.462527) knots 0 0 0 0 1 1 1 1
  spline S860 degree 3 poles (-13.474736, -44.462527) (-13.517986, -44.357669) (-13.558436, -44.251567) (-13.595774, -44.144531) knots 0 0 0 0 1 1 1 1
  spline S861 degree 3 poles (-13.595774, -44.144531) (-13.633112, -44.037184) (-13.667338, -43.929215) (-13.698454, -43.820001) knots 0 0 0 0 1 1 1 1
  spline S862 degree 3 poles (-13.698454, -43.820001) (-13.72988, -43.710788) (-13.757883, -43.600952) (-13.782775, -43.490182) knots 0 0 0 0 1 1 1 1
  spline S863 degree 3 poles (-13.782775, -43.490182) (-13.807667, -43.379413) (-13.829448, -43.268021) (-13.848117, -43.156007) knots 0 0 0 0 1 1 1 1
  spline S864 degree 3 poles (-13.848117, -43.156007) (-13.866786, -43.043993) (-13.882343, -42.931667) (-13.894478, -42.81872) knots 0 0 0 0 1 1 1 1
  spline S865 degree 3 poles (-13.894478, -42.81872) (-13.906613, -42.706083) (-13.915636, -42.592825) (-13.921548, -42.479566) knots 0 0 0 0 1 1 1 1
  spline S866 degree 3 poles (-13.921548, -42.479566) (-13.927459, -42.365996) (-13.929949, -42.252737) (-13.929331, -42.139168) knots 0 0 0 0 1 1 1 1
  spline S867 degree 3 poles (-13.929331, -42.139168) (-13.928694, -42.025598) (-13.924663, -41.912028) (-13.917818, -41.798769) knots 0 0 0 0 1 1 1 1
  spline S868 degree 3 poles (-13.917818, -41.798769) (-13.910665, -41.68551) (-13.900394, -41.572563) (-13.887014, -41.459926) knots 0 0 0 0 1 1 1 1
  spline S869 degree 3 poles (-13.887014, -41.459926) (-13.873324, -41.346979) (-13.856833, -41.234654) (-13.836909, -41.122934) knots 0 0 0 0 1 1 1 1
  spline S870 degree 3 poles (-13.836909, -41.122934) (-13.832873, -41.100237) (-13.826651, -41.078145) (-13.81824, -41.056659) knots 0 0 0 0 1 1 1 1
  spline S871 degree 3 poles (-13.81824, -41.056659) (-13.809538, -41.035206) (-13.79927, -41.01467) (-13.786814, -40.995051) knots 0 0 0 0 1 1 1 1
  spline S872 degree 3 poles (-13.786814, -40.995051) (-13.774378, -40.975777) (-13.760065, -40.95773) (-13.744187, -40.940911) knots 0 0 0 0 1 1 1 1
  spline S873 degree 3 poles (-13.744187, -40.940911) (-13.728016, -40.924126) (-13.710592, -40.90919) (-13.691602, -40.896105) knots 0 0 0 0 1 1 1 1
  spline S874 degree 3 poles (-13.691602, -40.896105) (-13.672943, -40.882743) (-13.652718, -40.871541) (-13.63155, -40.86219) knots 0 0 0 0 1 1 1 1
  spline S875 degree 3 poles (-13.63155, -40.86219) (-13.610402, -40.853183) (-13.588621, -40.846027) (-13.565897, -40.841031) knots 0 0 0 0 1 1 1 1
  spline S876 degree 3 poles (-13.565897, -40.841031) (-13.543504, -40.83607) (-13.52079, -40.833275) (-13.497757, -40.832942) knots 0 0 0 0 1 1 1 1
  spline S877 degree 3 poles (-13.497757, -40.832942) (-13.47443, -40.832322) (-13.451716, -40.834201) (-13.428991, -40.838231) knots 0 0 0 0 1 1 1 1
  line L15 (-2.355778, -42.81465) -> (-2.351422, -42.815287)
  spline S878 degree 3 poles (-2.351422, -42.815287) (-2.32902, -42.81966) (-2.306928, -42.826195) (-2.285148, -42.83489) knots 0 0 0 0 1 1 1 1
  spline S879 degree 3 poles (-2.285148, -42.83489) (-2.263989, -42.84393) (-2.243764, -42.854509) (-2.224473, -42.867266) knots 0 0 0 0 1 1 1 1
  spline S880 degree 3 poles (-2.224162, -42.866938) (-2.205493, -42.880024) (-2.187446, -42.894648) (-2.171266, -42.910828) knots 0 0 0 0 1 1 1 1
  spline S881 degree 3 poles (-2.170333, -42.910499) (-2.154775, -42.927318) (-2.140151, -42.945054) (-2.127394, -42.964034) knots 0 0 0 0 1 1 1 1
  spline S882 degree 3 poles (-2.127394, -42.964034) (-2.114326, -42.983326) (-2.103436, -43.00355) (-2.093479, -43.024691) knots 0 0 0 0 1 1 1 1
  spline S883 degree 3 poles (-2.093479, -43.024691) (-2.0857, -43.046178) (-2.078855, -43.06827) (-2.074187, -43.090672) knots 0 0 0 0 1 1 1 1
  spline S884 degree 3 poles (-2.074187, -43.090672) (-2.069831, -43.113386) (-2.067342, -43.136411) (-2.067342, -43.159437) knots 0 0 0 0 1 1 1 1
  spline S885 degree 3 poles (-2.067342, -43.159437) (-2.067342, -43.182462) (-2.06952, -43.205487) (-2.073876, -43.228201) knots 0 0 0 0 1 1 1 1
  spline S886 degree 3 poles (-2.073876, -43.228201) (-2.12086, -43.484277) (-2.184334, -43.736309) (-2.263989, -43.983985) knots 0 0 0 0 1 1 1 1
  spline S887 degree 3 poles (-2.263989, -43.983985) (-2.343332, -44.231972) (-2.438856, -44.473735) (-2.549625, -44.709276) knots 0 0 0 0 1 1 1 1
  spline S888 degree 3 poles (-2.549625, -44.709276) (-2.660395, -44.944817) (-2.786099, -45.172268) (-2.926428, -45.391629) knots 0 0 0 0 1 1 1 1
  spline S889 degree 3 poles (-2.926428, -45.391629) (-3.066757, -45.61099) (-3.220465, -45.820083) (-3.386931, -46.019513) knots 0 0 0 0 1 1 1 1
  spline S890 degree 3 poles (-3.386931, -46.019513) (-3.555263, -46.218977) (-3.734797, -46.406601) (-3.926465, -46.582712) knots 0 0 0 0 1 1 1 1
  spline S891 degree 3 poles (-3.925532, -46.582384) (-4.117823, -46.758823) (-4.32007, -46.921866) (-4.532897, -47.07184) knots 0 0 0 0 1 1 1 1
  spline S892 degree 3 poles (-4.532897, -47.07184) (-4.745413, -47.221504) (-4.966952, -47.357165) (-5.196269, -47.477874) knots 0 0 0 0 1 1 1 1
  spline S893 degree 3 poles (-5.196269, -47.477874) (-5.427454, -47.599551) (-5.66455, -47.705342) (-5.908492, -47.795576) knots 0 0 0 0 1 1 1 1
  spline S894 degree 3 poles (-5.908492, -47.795576) (-5.929961, -47.803666) (-5.952364, -47.809578) (-5.974145, -47.812672) knots 0 0 0 0 1 1 1 1
  spline S895 degree 3 poles (-5.974145, -47.812672) (-5.997792, -47.816737) (-6.020817, -47.817979) (-6.043842, -47.817048) knots 0 0 0 0 1 1 1 1
  spline S896 degree 3 poles (-6.04322, -47.81672) (-6.066867, -47.816117) (-6.089581, -47.813) (-6.111984, -47.807713) knots 0 0 0 0 1 1 1 1
  spline S897 degree 3 poles (-6.111362, -47.807074) (-6.134698, -47.802424) (-6.156168, -47.794956) (-6.177326, -47.784999) knots 0 0 0 0 1 1 1 1
  spline S898 degree 3 poles (-6.176392, -47.784671) (-6.198173, -47.775354) (-6.218086, -47.763841) (-6.236756, -47.75015) knots 0 0 0 0 1 1 1 1
  spline S899 degree 3 poles (-6.235822, -47.749822) (-6.255424, -47.736771) (-6.272538, -47.721525) (-6.288096, -47.704411) knots 0 0 0 0 1 1 1 1
  spline S900 degree 3 poles (-6.287473, -47.703772) (-6.303964, -47.687609) (-6.317655, -47.669251) (-6.32979, -47.649338) knots 0 0 0 0 1 1 1 1
  spline S901 degree 3 poles (-6.329166, -47.64901) (-6.341925, -47.629735) (-6.351882, -47.608888) (-6.359971, -47.587419) knots 0 0 0 0 1 1 1 1
  spline S902 degree 3 poles (-6.359971, -47.587419) (-6.367753, -47.565638) (-6.373662, -47.543547) (-6.377395, -47.520521) knots 0 0 0 0 1 1 1 1
  spline S903 degree 3 poles (-6.377395, -47.520521) (-6.38082, -47.497807) (-6.382374, -47.474782) (-6.381442, -47.451757) knots 0 0 0 0 1 1 1 1
  spline S904 degree 3 poles (-6.381442, -47.451757) (-6.380509, -47.428732) (-6.377395, -47.405707) (-6.371174, -47.382665) knots 0 0 0 0 1 1 1 1
  spline S905 degree 3 poles (-6.371174, -47.382665) (-6.366507, -47.360901) (-6.359039, -47.339121) (-6.349393, -47.317963) knots 0 0 0 0 1 1 1 1
  spline S906 degree 3 poles (-6.348771, -47.317634) (-6.339747, -47.297116) (-6.328234, -47.277202) (-6.314544, -47.258533) knots 0 0 0 0 1 1 1 1
  spline S907 degree 3 poles (-6.313922, -47.257894) (-6.300853, -47.239864) (-6.285607, -47.222751) (-6.268805, -47.206882) knots 0 0 0 0 1 1 1 1
  spline S908 degree 3 poles (-6.268805, -47.206882) (-6.251692, -47.191324) (-6.233334, -47.177323) (-6.213109, -47.164549) knots 0 0 0 0 1 1 1 1
  spline S909 degree 3 poles (-6.213109, -47.164549) (-6.194129, -47.153053) (-6.173594, -47.143096) (-6.151813, -47.135006) knots 0 0 0 0 1 1 1 1
  spline S910 degree 3 poles (-6.151813, -47.135006) (-5.714958, -46.973519) (-5.306106, -46.757892) (-4.925258, -46.487797) knots 0 0 0 0 1 1 1 1
  spline S911 degree 3 poles (-4.925258, -46.487797) (-4.645224, -46.288366) (-4.386346, -46.063094) (-4.148939, -45.812929) knots 0 0 0 0 1 1 1 1
  spline S912 degree 3 poles (-4.148626, -45.812289) (-3.911842, -45.562764) (-3.700571, -45.292374) (-3.515126, -45.001449) knots 0 0 0 0 1 1 1 1
  spline S913 degree 3 poles (-3.514813, -45.001121) (-3.32968, -44.710523) (-3.173794, -44.404662) (-3.047156, -44.083867) knots 0 0 0 0 1 1 1 1
  spline S914 degree 3 poles (-3.047154, -44.083538) (-2.920517, -43.763071) (-2.825617, -43.43294) (-2.762452, -43.093769) knots 0 0 0 0 1 1 1 1
  spline S915 degree 3 poles (-2.762452, -43.093769) (-2.758097, -43.071383) (-2.751563, -43.049603) (-2.743161, -43.028406) knots 0 0 0 0 1 1 1 1
  spline S916 degree 3 poles (-2.743161, -43.028406) (-2.73445, -43.006975) (-2.72387, -42.987062) (-2.711424, -42.96777) knots 0 0 0 0 1 1 1 1
  spline S917 degree 3 poles (-2.711423, -42.967732) (-2.698667, -42.94879) (-2.684354, -42.931055) (-2.668486, -42.914564) knots 0 0 0 0 1 1 1 1
  spline S918 degree 3 poles (-2.668485, -42.914525) (-2.652617, -42.898384) (-2.635193, -42.88376) (-2.616213, -42.870692) knots 0 0 0 0 1 1 1 1
  spline S919 degree 3 poles (-2.616211, -42.870653) (-2.597232, -42.857934) (-2.577319, -42.846733) (-2.556472, -42.83771) knots 0 0 0 0 1 1 1 1
  spline S920 degree 3 poles (-2.55647, -42.837671) (-2.535313, -42.828686) (-2.513844, -42.821841) (-2.491441, -42.816863) knots 0 0 0 0 1 1 1 1
  spline S921 degree 3 poles (-2.49144, -42.816824) (-2.469038, -42.812195) (-2.446636, -42.809709) (-2.42361, -42.809089) knots 0 0 0 0 1 1 1 1
  spline S922 degree 3 poles (-2.423609, -42.80905) (-2.400897, -42.80877) (-2.378183, -42.810642) (-2.35578, -42.814689) knots 0 0 0 0 1 1 1 1
  spline S923 degree 3 poles (-2.297282, -39.607019) (-2.282347, -39.609504) (-2.267412, -39.61324) (-2.253099, -39.617909) knots 0 0 0 0 1 1 1 1
  spline S924 degree 3 poles (-2.253099, -39.617909) (-2.238475, -39.622577) (-2.224162, -39.627866) (-2.210471, -39.6344) knots 0 0 0 0 1 1 1 1
  spline S925 degree 3 poles (-2.210471, -39.6344) (-2.19647, -39.640932) (-2.18309, -39.648402) (-2.170333, -39.656492) knots 0 0 0 0 1 1 1 1
  spline S926 degree 3 poles (-2.170333, -39.656492) (-2.157265, -39.664582) (-2.14513, -39.673605) (-2.133306, -39.683562) knots 0 0 0 0 1 1 1 1
  spline S927 degree 3 poles (-2.133306, -39.683562) (-2.121793, -39.693208) (-2.110592, -39.703787) (-2.100324, -39.714988) knots 0 0 0 0 1 1 1 1
  spline S928 degree 3 poles (-2.100324, -39.714988) (-2.090056, -39.726501) (-2.08041, -39.738325) (-2.071698, -39.750771) knots 0 0 0 0 1 1 1 1
  spline S929 degree 3 poles (-2.071698, -39.750771) (-2.062675, -39.763217) (-2.054896, -39.776285) (-2.04774, -39.789976) knots 0 0 0 0 1 1 1 1
  spline S930 degree 3 poles (-2.04774, -39.789976) (-2.040584, -39.803355) (-2.03436, -39.817357) (-2.029071, -39.83167) knots 0 0 0 0 1 1 1 1
  spline S931 degree 3 poles (-2.029071, -39.83167) (-2.024092, -39.845983) (-2.019736, -39.860607) (-2.016314, -39.875542) knots 0 0 0 0 1 1 1 1
  spline S932 degree 3 poles (-2.016314, -39.875542) (-2.012891, -39.890477) (-2.010402, -39.905723) (-2.009157, -39.92097) knots 0 0 0 0 1 1 1 1
  spline S933 degree 3 poles (-2.009157, -39.92097) (-2.007602, -39.936216) (-2.00729, -39.951463) (-2.007912, -39.966709) knots 0 0 0 0 1 1 1 1
  spline S934 degree 3 poles (-2.007912, -39.966709) (-2.008534, -39.981955) (-2.01009, -39.997202) (-2.012579, -40.012137) knots 0 0 0 0 1 1 1 1
  spline S935 degree 3 poles (-2.012579, -40.012137) (-2.015069, -40.027383) (-2.018491, -40.042007) (-2.023159, -40.056631) knots 0 0 0 0 1 1 1 1
  spline S936 degree 3 poles (-2.023159, -40.056631) (-2.027515, -40.071255) (-2.033115, -40.085568) (-2.039338, -40.09957) knots 0 0 0 0 1 1 1 1
  spline S937 degree 3 poles (-2.039338, -40.09957) (-2.045873, -40.113572) (-2.053029, -40.126951) (-2.061119, -40.14002) knots 0 0 0 0 1 1 1 1
  spline S938 degree 3 poles (-2.061119, -40.14002) (-2.069209, -40.152777) (-2.077921, -40.165223) (-2.087878, -40.177046) knots 0 0 0 0 1 1 1 1
  line L16 (-2.087878, -40.177046) -> (-2.343954, -40.488819)
  spline S939 degree 3 poles (-2.343954, -40.488819) (-2.611232, -40.840419) (-2.836816, -41.217222) (-3.021017, -41.618606) knots 0 0 0 0 1 1 1 1
  spline S940 degree 3 poles (-3.021017, -41.618606) (-3.205218, -42.01999) (-3.34368, -42.43662) (-3.436403, -42.868496) knots 0 0 0 0 1 1 1 1
  spline S941 degree 3 poles (-3.436403, -42.868496) (-3.486498, -43.171868) (-3.565841, -43.467772) (-3.674433, -43.755897) knots 0 0 0 0 1 1 1 1
  spline S942 degree 3 poles (-3.674433, -43.755897) (-3.782713, -44.043711) (-3.918375, -44.318457) (-4.081106, -44.579512) knots 0 0 0 0 1 1 1 1
  spline S943 degree 3 poles (-4.081106, -44.579512) (-4.243527, -44.840878) (-4.430217, -45.083575) (-4.641177, -45.308539) knots 0 0 0 0 1 1 1 1
  spline S944 degree 3 poles (-4.641177, -45.308539) (-4.851203, -45.532254) (-5.081454, -45.733879) (-5.33162, -45.912793) knots 0 0 0 0 1 1 1 1
  spline S945 degree 3 poles (-5.33162, -45.912793) (-5.577428, -46.087657) (-5.83786, -46.236387) (-6.113229, -46.359294) knots 0 0 0 0 1 1 1 1
  spline S946 degree 3 poles (-6.113229, -46.359294) (-6.388908, -46.481885) (-6.67361, -46.576163) (-6.967959, -46.641818) knots 0 0 0 0 1 1 1 1
  spline S947 degree 3 poles (-6.967959, -46.641818) (-7.261996, -46.707469) (-7.559766, -46.743562) (-7.861272, -46.749476) knots 0 0 0 0 1 1 1 1
  spline S948 degree 3 poles (-7.861272, -46.749476) (-8.162464, -46.755383) (-8.461479, -46.731738) (-8.758007, -46.677601) knots 0 0 0 0 1 1 1 1
  spline S949 degree 3 poles (-8.758007, -46.677601) (-8.918248, -46.648972) (-9.076625, -46.611946) (-9.232822, -46.566209) knots 0 0 0 0 1 1 1 1
  spline S950 degree 3 poles (-9.232822, -46.566209) (-9.38902, -46.520779) (-9.542417, -46.46695) (-9.693013, -46.404722) knots 0 0 0 0 1 1 1 1
  spline S951 degree 3 poles (-9.693013, -46.404722) (-9.84361, -46.342801) (-9.990473, -46.272792) (-10.133602, -46.195007) knots 0 0 0 0 1 1 1 1
  spline S952 degree 3 poles (-10.133602, -46.195007) (-10.27642, -46.117217) (-10.414882, -46.032273) (-10.548988, -45.93955) knots 0 0 0 0 1 1 1 1
  spline S953 degree 3 poles (-10.548988, -45.939241) (-10.682782, -45.847138) (-10.811599, -45.74757) (-10.934814, -45.641157) knots 0 0 0 0 1 1 1 1
  spline S954 degree 3 poles (-10.934814, -45.640848) (-11.05803, -45.534743) (-11.175335, -45.422418) (-11.286725, -45.303247) knots 0 0 0 0 1 1 1 1
  spline S955 degree 3 poles (-11.286725, -45.302939) (-11.398117, -45.184388) (-11.502664, -45.059928) (-11.600676, -44.929867) knots 0 0 0 0 1 1 1 1
  spline S956 degree 3 poles (-11.600676, -44.929247) (-11.698687, -44.799806) (-11.789544, -44.664767) (-11.873243, -44.525061) knots 0 0 0 0 1 1 1 1
  spline S957 degree 3 poles (-11.872932, -44.52413) (-11.886001, -44.505147) (-11.89658, -44.4843) (-11.905292, -44.462208) knots 0 0 0 0 1 1 1 1
  spline S958 degree 3 poles (-11.904981, -44.461588) (-11.913693, -44.440117) (-11.919916, -44.417714) (-11.923961, -44.394377) knots 0 0 0 0 1 1 1 1
  spline S959 degree 3 poles (-11.923961, -44.393758) (-11.928007, -44.371041) (-11.929872, -44.347705) (-11.929251, -44.324058) knots 0 0 0 0 1 1 1 1
  spline S960 degree 3 poles (-11.928939, -44.323438) (-11.928318, -44.30041) (-11.925514, -44.277074) (-11.920227, -44.254049) knots 0 0 0 0 1 1 1 1
  spline S961 degree 3 poles (-11.919916, -44.253429) (-11.914628, -44.231024) (-11.907159, -44.208932) (-11.897202, -44.187463) knots 0 0 0 0 1 1 1 1
  spline S962 degree 3 poles (-11.897202, -44.186843) (-11.887556, -44.165993) (-11.875731, -44.145768) (-11.861731, -44.126477) knots 0 0 0 0 1 1 1 1
  spline S963 degree 3 poles (-11.86142, -44.125857) (-11.847729, -44.107497) (-11.832172, -44.090073) (-11.814747, -44.074204) knots 0 0 0 0 1 1 1 1
  spline S964 degree 3 poles (-11.814436, -44.073273) (-11.797323, -44.058024) (-11.778343, -44.044022) (-11.758118, -44.031887) knots 0 0 0 0 1 1 1 1
  spline S965 degree 3 poles (-11.758118, -44.031268) (-11.737893, -44.019753) (-11.716734, -44.009796) (-11.694643, -44.002017) knots 0 0 0 0 1 1 1 1
  spline S966 degree 3 poles (-11.694332, -44.001397) (-11.67224, -43.994236) (-11.649526, -43.988638) (-11.62619, -43.985215) knots 0 0 0 0 1 1 1 1
  spline S967 degree 3 poles (-11.625879, -43.984595) (-11.602854, -43.982101) (-11.579206, -43.981167) (-11.55587, -43.982731) knots 0 0 0 0 1 1 1 1
  spline S968 degree 3 poles (-11.555559, -43.981792) (-11.532223, -43.983973) (-11.509198, -43.98802) (-11.486173, -43.993932) knots 0 0 0 0 1 1 1 1
  spline S969 degree 3 poles (-11.486173, -43.993305) (-11.463459, -44.000153) (-11.441678, -44.008556) (-11.42052, -44.019135) knots 0 0 0 0 1 1 1 1
  spline S970 degree 3 poles (-11.42052, -44.018508) (-11.399362, -44.029714) (-11.379448, -44.04216) (-11.36109, -44.056784) knots 0 0 0 0 1 1 1 1
  spline S971 degree 3 poles (-11.360779, -44.056157) (-11.342421, -44.071408) (-11.325619, -44.087588) (-11.310373, -44.105635) knots 0 0 0 0 1 1 1 1
  spline S972 degree 3 poles (-11.310061, -44.104697) (-11.294815, -44.12337) (-11.281436, -44.142662) (-11.270234, -44.163509) knots 0 0 0 0 1 1 1 1
  spline S973 degree 3 poles (-11.269923, -44.162571) (-11.12835, -44.400605) (-10.962818, -44.620277) (-10.77395, -44.821903) knots 0 0 0 0 1 1 1 1